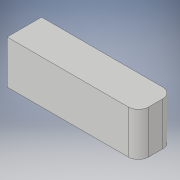
# Autodesk Inventor part: Battery
Saved by Autodesk Inventor 2019 (Build 230136000, 136)
## iProperties
Created: 2018-12-25
Part Number: Battery
Material: Generic
Document SubType Name: Modeling
Designer: Martin
Density: 1 g/cm^3
Appearance: Default
Author: Martin
Autodesk Inventor part; units mm, degrees
ref_plane "YZ Plane" through (0, 0, 0) normal (1, 0, 0) x (0, 1, 0)
ref_plane "XZ Plane" through (0, 0, 0) normal (0, 1, 0) x (-1, 0, 0)
ref_plane "XY Plane" through (0, 0, 0) normal (0, 0, 1) x (1, 0, 0)
sketch "Sketch1" plane through (0, 0, 0) normal (0, 0, 1) x (1, 0, 0)
  line L0 (51.5, -17) -> (-51.5, -17)
  line L1 (-51.5, -17) -> (-51.5, 17)
  line L2 (-51.5, 17) -> (51.5, 17)
  line L3 (51.5, 17) -> (51.5, -17)
  line L4 (51.5, -17) -> (-51.5, 17) construction
  line L5 (-51.5, -17) -> (51.5, 17) construction
  point P0 (0, 0)
  dimension "d0" = 103
  dimension "d1" = 34
  constraints: 12 end point, 2 midpoint, 2 parallel, 1 horizontal, 1 perpendicular
  measures "d0" distance of L1.end L2.end
  measures "d1" distance of L0.end L1.end
extrude "Extrusion1" add sketch "Sketch1" along normal blind 27
fillet "Fillet1" radius 8 2 edges at (51.5, 0, 27) (51.5, 0, 0)
body "Solid1"
